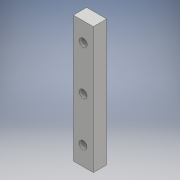
# Autodesk Inventor part: slider-rail
Saved by Autodesk Inventor 2018 (Build 220112000, 112)
## iProperties
Created: 2025-02-27
Part Number: slider-rail
Material: Generic
Document SubType Name: Modeling
Designer: neo
Density: 1 g/cm^3
Appearance: Default
Author: neo
Autodesk Inventor part; units mm, degrees
ref_plane "YZ Plane" through (0, 0, 0) normal (1, 0, 0) x (0, 1, 0)
ref_plane "XZ Plane" through (0, 0, 0) normal (0, 1, 0) x (-1, 0, 0)
ref_plane "XY Plane" through (0, 0, 0) normal (0, 0, 1) x (1, 0, 0)
sketch "Sketch1" plane through (0, 0, 0) normal (0, 0, 1) x (1, 0, 0)
  line L0 (4.6071, -2.8259) -> (-4.3929, -2.8259)
  line L1 (-4.3929, -2.8259) -> (-4.3929, 3.1741)
  line L2 (-4.3929, 3.1741) -> (4.6071, 3.1741)
  line L3 (4.6071, 3.1741) -> (4.6071, -2.8259)
  point P0 (0, 0)
  dimension "d0" = 9
  dimension "d1" = 6
  constraints: 8 end point, 2 parallel, 1 horizontal, 1 perpendicular
  measures "d0" distance of L1.end L2.end
  measures "d1" distance of L2.end L0.start
extrude "Extrusion1" add sketch "Sketch1" along normal blind 57
sketch "Sketch2" plane through (-4.3929, 3.1741, 0) normal (0, 1, 0) x (1, 0, 0)
  line L0 (0, 0) -> (9, 0) projected
  line L1 (0, 0) -> (0, -57) projected
  line L2 (9, -57) -> (0, -57) projected
  line L3 (9, 0) -> (9, -57) projected
  line L4 (-2.9131, -28.5) -> (15.4584, -28.5)
  line L5 (4.5, -57) -> (4.3929, 0)
  circle A0 centre (4.484, -48.5) radius 1.75
  circle A1 centre (4.4464, -28.5) radius 1.75
  circle A2 centre (4.4088, -8.5001) radius 1.75
  dimension "d4" = 3.5
  dimension "d5" = 40
  dimension "d6" = 8.5
  dimension "d9" = 20
  constraints: 4 end point, 3 centre point, 1 horizontal, 1 midpoint, 1 point on line, 5 other
  measures "d4" diameter of A0
  measures "d5" diameter of A0.centre L4
  measures "d6" distance from line of L2 A0.centre
  measures "d9" distance of A0.centre A1.centre
hole "Hole1" at (0.0912, 3.1741, 48.5) at (0.0536, 3.1741, 28.5) at (0.016, 3.1741, 8.5001) direction (0, -1, 0) diameter 3.5 end through all counterbore diameter 6 counterbore depth 3.5
body "Solid1"
